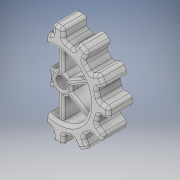
# Autodesk Inventor part: GearCasing
Saved by Autodesk Inventor 2017 (Build 210142000, 142)
## iProperties
Created: 2017-01-26
Part Number: GearCasing
Material: Generic
Document SubType Name: Modeling
Designer: Moonlight.Admin
Density: 1 g/cm^3
Appearance: Default
Author: Moonlight.Admin
Autodesk Inventor part; units mm, degrees
ref_plane "YZ Plane" through (0, 0, 0) normal (1, 0, 0) x (0, 1, 0)
ref_plane "XZ Plane" through (0, 0, 0) normal (0, 1, 0) x (-1, 0, 0)
ref_plane "XY Plane" through (0, 0, 0) normal (0, 0, 1) x (1, 0, 0)
sketch "Sketch2" plane through (0, 0, 0) normal (0, 0, 1) x (1, 0, 0)
  circle A0 centre (0, 0) radius 50.8
  line L0 (-8.0763, 82.55) -> (8.0763, 82.55)
  line L1 (8.0763, 82.55) -> (9.525, 65.9911)
  line L2 (-9.525, 65.9911) -> (-8.0763, 82.55)
  line L3 (0, 0) -> (0, 31.3824) construction
  line L4 (-41.2445, 52.3875) -> (-48.2693, 67.4523)
  line L5 (-48.2693, 67.4523) -> (-34.2807, 75.5285)
  line L6 (-34.2807, 75.5285) -> (-24.7467, 61.9125)
  line L7 (0, 0) -> (-15.6912, 27.1779) construction
  line L8 (-61.9125, 24.7467) -> (-75.5285, 34.2807)
  line L9 (-75.5285, 34.2807) -> (-67.4523, 48.2693)
  line L10 (-67.4523, 48.2693) -> (-52.3875, 41.2445)
  line L11 (0, 0) -> (-27.1779, 15.6912) construction
  line L12 (-65.9911, -9.525) -> (-82.55, -8.0763)
  line L13 (-82.55, -8.0763) -> (-82.55, 8.0763)
  line L14 (-82.55, 8.0763) -> (-65.9911, 9.525)
  line L15 (0, 0) -> (-31.3824, 0) construction
  line L16 (-52.3875, -41.2445) -> (-67.4523, -48.2693)
  line L17 (-67.4523, -48.2693) -> (-75.5285, -34.2807)
  line L18 (-75.5285, -34.2807) -> (-61.9125, -24.7467)
  line L19 (0, 0) -> (-27.1779, -15.6912) construction
  line L20 (-24.7467, -61.9125) -> (-34.2807, -75.5285)
  line L21 (-34.2807, -75.5285) -> (-48.2693, -67.4523)
  line L22 (-48.2693, -67.4523) -> (-41.2445, -52.3875)
  line L23 (0, 0) -> (-15.6912, -27.1779) construction
  line L24 (9.525, -65.9911) -> (8.0763, -82.55)
  line L25 (8.0763, -82.55) -> (-8.0763, -82.55)
  line L26 (-8.0763, -82.55) -> (-9.525, -65.9911)
  line L27 (0, 0) -> (0, -31.3824) construction
  line L28 (41.2445, -52.3875) -> (48.2693, -67.4523)
  line L29 (48.2693, -67.4523) -> (34.2807, -75.5285)
  line L30 (34.2807, -75.5285) -> (24.7467, -61.9125)
  line L31 (0, 0) -> (15.6912, -27.1779) construction
  line L32 (61.9125, -24.7467) -> (75.5285, -34.2807)
  line L33 (75.5285, -34.2807) -> (67.4523, -48.2693)
  line L34 (67.4523, -48.2693) -> (52.3875, -41.2445)
  line L35 (0, 0) -> (27.1779, -15.6912) construction
  line L36 (65.9911, 9.525) -> (82.55, 8.0763)
  line L37 (82.55, 8.0763) -> (82.55, -8.0763)
  line L38 (82.55, -8.0763) -> (65.9911, -9.525)
  line L39 (0, 0) -> (31.3824, 0) construction
  line L40 (52.3875, 41.2445) -> (67.4523, 48.2693)
  line L41 (67.4523, 48.2693) -> (75.5285, 34.2807)
  line L42 (75.5285, 34.2807) -> (61.9125, 24.7467)
  line L43 (0, 0) -> (27.1779, 15.6912) construction
  line L44 (24.7467, 61.9125) -> (34.2807, 75.5285)
  line L45 (34.2807, 75.5285) -> (48.2693, 67.4523)
  line L46 (48.2693, 67.4523) -> (41.2445, 52.3875)
  line L47 (0, 0) -> (15.6912, 27.1779) construction
  arc A1 (24.7467, 61.9125) -> (9.525, 65.9911) centre (0, 0) ccw
  arc A2 (52.3875, 41.2445) -> (41.2445, 52.3875) centre (0, 0) ccw
  arc A3 (65.9911, 9.525) -> (61.9125, 24.7467) centre (0, 0) ccw
  arc A4 (61.9125, -24.7467) -> (65.9911, -9.525) centre (0, 0) ccw
  arc A5 (41.2445, -52.3875) -> (52.3875, -41.2445) centre (0, 0) ccw
  arc A6 (9.525, -65.9911) -> (24.7467, -61.9125) centre (0, 0) ccw
  arc A7 (-24.7467, -61.9125) -> (-9.525, -65.9911) centre (0, 0) ccw
  arc A8 (-52.3875, -41.2445) -> (-41.2445, -52.3875) centre (0, 0) ccw
  arc A9 (-65.9911, -9.525) -> (-61.9125, -24.7467) centre (0, 0) ccw
  arc A10 (-61.9125, 24.7467) -> (-65.9911, 9.525) centre (0, 0) ccw
  arc A11 (-9.525, 65.9911) -> (-24.7467, 61.9125) centre (0, 0) ccw
  arc A12 (-41.2445, 52.3875) -> (-52.3875, 41.2445) centre (0, 0) ccw
  line L48 (12.7, 25.4) -> (-12.7, 25.4) construction
  line L49 (-12.7, 25.4) -> (-12.7, -25.4) construction
  line L50 (-12.7, -25.4) -> (12.7, -25.4) construction
  line L51 (12.7, -25.4) -> (12.7, 25.4) construction
  line L52 (-12.7, 18.75) -> (-57.2, 18.75) construction
  line L53 (-57.2, 18.75) -> (-57.2, -18.75) construction
  line L54 (-57.2, -18.75) -> (-12.7, -18.75) construction
  line L55 (-12.7, -18.75) -> (-12.7, 18.75) construction
  point P0 (0, 82.55)
  point P1 (-41.275, 71.4904)
  point P2 (-71.4904, 41.275)
  point P3 (-82.55, 0)
  point P4 (-71.4904, -41.275)
  point P5 (-41.275, -71.4904)
  point P6 (0, -82.55)
  point P7 (41.275, -71.4904)
  point P8 (71.4904, -41.275)
  point P9 (82.55, 0)
  point P10 (71.4904, 41.275)
  point P11 (41.275, 71.4904)
  dimension "d6" = 101.6
  dimension "d11" = 10
  dimension "d13" = 19.05
  dimension "d16" = 360
  dimension "d18" = 165.1
  dimension "d19" = 66.675
  dimension "d47" = 25.4
  dimension "d48" = 50.8
  dimension "d49" = 12.7
  dimension "d50" = 25.4
  dimension "d51" = 44.5
  dimension "d52" = 37.5
  dimension "d53" = 18.75
  constraints: 112 end point, 24 point on circle, 13 centre point, 13 point on line, 4 parallel, 3 perpendicular, 2 coincident, 2 horizontal, 1 equal length, 1 midpoint, 1 vertical, 133 other
  measures "d6" diameter of A0
  measures "d11" angle of L1 L2
  measures "d13" distance of L1.end L2.start
  measures "d18" distance between parallel lines of L25 L0
  measures "d19" radius of A1
  measures "d47" distance of L48.start L48.end
  measures "d48" distance of L48.end L49.end
  measures "d49" distance from line of point (0, 0) L51
  measures "d50" distance from line of point (0, 0) L48
  measures "d51" distance of L52.start L52.end
  measures "d52" distance of L52.end L53.end
  measures "d53" distance from line of point (0, 0) L52
extrude "Extrusion1" add sketch "Sketch2" along normal blind 38.1
fillet "Fillet1" radius 4.7625 96 edges at (0, 82.55, 38.1) (-8.8006, 74.2706, 38.1) (-17.2568, 64.4031, 38.1) (-29.5137, 68.7205, 38.1) (-41.275, 71.4904, 38.1) (-44.7569, 59.9199, 38.1) (-47.1463, 47.1463, 38.1) (-59.9199, 44.7569, 38.1) (-71.4904, 41.275, 38.1) (-68.7205, 29.5137, 38.1) (-64.4031, 17.2568, 38.1) (-74.2706, 8.8006, 38.1) (-82.55, 0, 38.1) (-74.2706, -8.8006, 38.1) (-64.4031, -17.2568, 38.1) (-68.7205, -29.5137, 38.1) (-71.4904, -41.275, 38.1) (-59.9199, -44.7569, 38.1) (-47.1463, -47.1463, 38.1) (-44.7569, -59.9199, 38.1) (-41.275, -71.4904, 38.1) (-29.5137, -68.7205, 38.1) (-17.2568, -64.4031, 38.1) (-8.8006, -74.2706, 38.1) (0, -82.55, 38.1) (8.8006, -74.2706, 38.1) (17.2568, -64.4031, 38.1) (29.5137, -68.7205, 38.1) (41.275, -71.4904, 38.1) (44.7569, -59.9199, 38.1) (47.1463, -47.1463, 38.1) (59.9199, -44.7569, 38.1) (71.4904, -41.275, 38.1) (68.7205, -29.5137, 38.1) (64.4031, -17.2568, 38.1) (74.2706, -8.8006, 38.1) (82.55, 0, 38.1) (74.2706, 8.8006, 38.1) (64.4031, 17.2568, 38.1) (68.7205, 29.5137, 38.1) (71.4904, 41.275, 38.1) (59.9199, 44.7569, 38.1) (47.1463, 47.1463, 38.1) (44.7569, 59.9199, 38.1) (41.275, 71.4904, 38.1) (29.5137, 68.7205, 38.1) (17.2568, 64.4031, 38.1) (8.8006, 74.2706, 38.1) (8.0763, -82.55, 19.05) (-8.0763, -82.55, 19.05) (9.525, -65.9911, 19.05) (24.7467, -61.9125, 19.05) (34.2807, -75.5285, 19.05) (48.2693, -67.4523, 19.05) (41.2445, -52.3875, 19.05) (52.3875, -41.2445, 19.05) (67.4523, -48.2693, 19.05) (75.5285, -34.2807, 19.05) (65.9911, -9.525, 19.05) (82.55, -8.0763, 19.05) (82.55, 8.0763, 19.05) (61.9125, -24.7467, 19.05) (61.9125, 24.7467, 19.05) (75.5285, 34.2807, 19.05) (67.4523, 48.2693, 19.05) (65.9911, 9.525, 19.05) (52.3875, 41.2445, 19.05) (41.2445, 52.3875, 19.05) (48.2693, 67.4523, 19.05) (34.2807, 75.5285, 19.05) (24.7467, 61.9125, 19.05) (9.525, 65.9911, 19.05) (8.0763, 82.55, 19.05) (-8.0763, 82.55, 19.05) (-9.525, 65.9911, 19.05) (-24.7467, 61.9125, 19.05) (-34.2807, 75.5285, 19.05) (-48.2693, 67.4523, 19.05) (-41.2445, 52.3875, 19.05) (-52.3875, 41.2445, 19.05) (-67.4523, 48.2693, 19.05) (-75.5285, 34.2807, 19.05) (-61.9125, 24.7467, 19.05) (-65.9911, 9.525, 19.05) (-82.55, 8.0763, 19.05) (-82.55, -8.0763, 19.05) (-65.9911, -9.525, 19.05) (-61.9125, -24.7467, 19.05) (-75.5285, -34.2807, 19.05) (-67.4523, -48.2693, 19.05) (-52.3875, -41.2445, 19.05) (-41.2445, -52.3875, 19.05) (-48.2693, -67.4523, 19.05) (-34.2807, -75.5285, 19.05) (-24.7467, -61.9125, 19.05) (-9.525, -65.9911, 19.05)
fillet "Fillet2" radius 4.7625 1 edges at (-50.8, 0, 38.1)
sketch "Sketch3" plane through (0, 0, 0) normal (0, 0, -1) x (-1, 0, 0)
  circle A0 centre (0, 0) radius 50.8 construction
  line L0 (-4.7625, 16.8005) -> (-4.7625, 53.7645)
  line L1 (4.7625, 16.8005) -> (4.7625, 53.7645)
  circle A1 centre (0, 0) radius 9.525
  line L2 (-16.9309, 4.2758) -> (-48.9427, 22.7578)
  line L3 (-12.1684, 12.5247) -> (-44.1802, 31.0067)
  line L4 (-12.1684, -12.5247) -> (-44.1802, -31.0067)
  line L5 (-16.9309, -4.2758) -> (-48.9427, -22.7578)
  line L6 (4.7625, -16.8005) -> (4.7625, -53.7645)
  line L7 (-4.7625, -16.8005) -> (-4.7625, -53.7645)
  line L8 (16.9309, -4.2758) -> (48.9427, -22.7578)
  line L9 (12.1684, -12.5247) -> (44.1802, -31.0067)
  line L10 (12.1684, 12.5247) -> (44.1802, 31.0067)
  line L11 (16.9309, 4.2758) -> (48.9427, 22.7578)
  arc A2 (4.7625, 53.7645) -> (-4.7625, 53.7645) centre (0, 0) ccw
  arc A3 (48.9427, 22.7578) -> (44.1802, 31.0067) centre (0, 0) ccw
  arc A4 (44.1802, -31.0067) -> (48.9427, -22.7578) centre (0, 0) ccw
  arc A5 (-4.7625, -53.7645) -> (4.7625, -53.7645) centre (0, 0) ccw
  arc A6 (-44.1802, 31.0067) -> (-48.9427, 22.7578) centre (0, 0) ccw
  arc A7 (-48.9427, -22.7578) -> (-44.1802, -31.0067) centre (0, 0) ccw
  arc A8 (12.1684, 12.5247) -> (4.7625, 16.8005) centre (0, 0) ccw
  arc A9 (16.9309, -4.2758) -> (16.9309, 4.2758) centre (0, 0) ccw
  arc A10 (4.7625, -16.8005) -> (12.1684, -12.5247) centre (0, 0) ccw
  arc A11 (-12.1684, -12.5247) -> (-4.7625, -16.8005) centre (0, 0) ccw
  arc A12 (-4.7625, 16.8005) -> (-12.1684, 12.5247) centre (0, 0) ccw
  arc A13 (-16.9309, 4.2758) -> (-16.9309, -4.2758) centre (0, 0) ccw
  dimension "d27" = 101.6
  dimension "d30" = 9.525
  dimension "d31" = 4.7625
  dimension "d32" = 19.05
  dimension "d35" = 360
  dimension "d37" = 53.975
  dimension "d38" = 17.4625
  constraints: 24 end point, 24 point on circle, 13 centre point, 3 coincident, 1 parallel, 1 vertical, 37 other
  measures "d27" diameter of A0
  measures "d30" distance between parallel lines of L1 L0
  measures "d31" distance from line of point (0, 0) L1
  measures "d32" diameter of A1
  measures "d37" radius of A2
  measures "d38" radius of A8
extrude "Extrusion2" add sketch "Sketch3" against normal blind 33.3375
fillet "Fillet3" radius 3.175 19 edges at (-31.5563, 12.7198, 33.3375) (-17.4625, 0, 33.3375) (-31.5563, -12.7198, 33.3375) (-26.7938, -20.9686, 33.3375) (-8.7312, -15.123, 33.3375) (-4.7625, -33.6884, 33.3375) (4.7625, -33.6884, 33.3375) (8.7313, -15.123, 33.3375) (26.7938, -20.9686, 33.3375) (31.5563, -12.7198, 33.3375) (17.4625, 0, 33.3375) (31.5563, 12.7198, 33.3375) (26.7938, 20.9686, 33.3375) (8.7312, 15.123, 33.3375) (4.7625, 33.6884, 33.3375) (-4.7625, 33.6884, 33.3375) (-8.7313, 15.123, 33.3375) (-26.7938, 20.9686, 33.3375) (9.525, 0, 33.3375)
sketch "Sketch5" plane through (0, 0, 0) normal (0, 0, -1) x (-1, 0, 0)
  line L0 (15.875, 85.1649) -> (143.094, 85.1649)
  line L1 (143.094, 85.1649) -> (143.094, -83.0513)
  line L2 (143.094, -83.0513) -> (15.875, -83.0513)
  line L3 (15.875, -83.0513) -> (15.875, 85.1649)
  point P0 (0, 0)
  dimension "d43" = 15.875
  constraints: 8 end point, 2 parallel, 1 horizontal, 1 perpendicular
  measures "d43" distance from line of L3 point (0, 0)
extrude "Extrusion4" cut sketch "Sketch5" against normal through all
shell "Shell1" [suppressed]
sketch "Sketch4" plane through (0, 0, 0) normal (0, 0, -1) x (-1, 0, 0)
  circle A0 centre (0, 0) radius 57.15
  dimension "d46" = 114.3
  constraints: 1 centre point, 1 coincident
  measures "d46" diameter of A0
extrude "Extrusion3" [suppressed]
equation "\"d31\" = 0.5 * d30"
body "Solid1"
